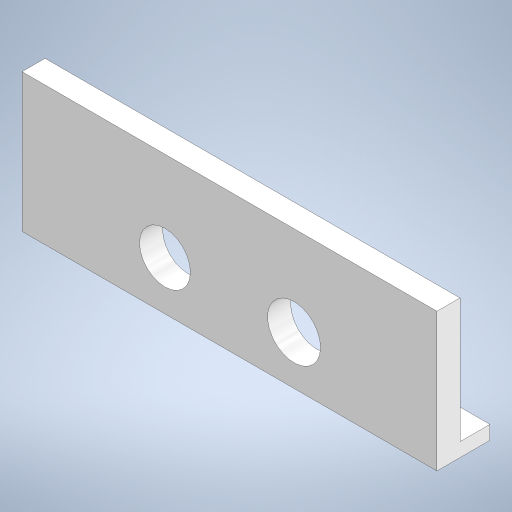
# Autodesk Inventor part: wall
Saved by Autodesk Inventor 2024 (Build 280153000, 153)
## iProperties
Created: 2023-08-11
Part Number: wall
Material: ABS Plastic
Document SubType Name: Modeling
Designer: l1534
Density: 1.06 g/cm^3
Appearance: Smooth - White
Author: l1534
Autodesk Inventor part; units mm, degrees
ref_plane "YZ Plane" through (0, 0, 0) normal (1, 0, 0) x (0, 1, 0)
ref_plane "XZ Plane" through (0, 0, 0) normal (0, 1, 0) x (-1, 0, 0)
ref_plane "XY Plane" through (0, 0, 0) normal (0, 0, 1) x (1, 0, 0)
sketch "Sketch1" plane through (0, 0, 0) normal (0, 0, 1) x (1, 0, 0)
  line L0 (-96.9802, 31.1578) -> (83.0198, 31.1578)
  line L1 (83.0198, 31.1578) -> (83.0198, -28.8422)
  line L2 (83.0198, -28.8422) -> (-96.9802, -28.8422)
  line L3 (-96.9802, -28.8422) -> (-96.9802, 31.1578)
  point P0 (0, 0)
  dimension "d0" = 180
  dimension "d1" = 60
  constraints: 8 end point, 2 parallel, 1 horizontal, 1 perpendicular
  measures "d0" distance of L0.start L0.end
  measures "d1" distance of L0.end L1.end
extrude "Extrusion1" add sketch "Sketch1" along normal blind 10
sketch "Sketch4" plane through (0, 0, 0) normal (0, 0, -1) x (-1, 0, 0)
  circle A0 centre (-21.0198, -7.6922) radius 11.5
  line L0 (96.9802, -28.8422) -> (-83.0198, -28.8422) projected
  line L1 (-83.0198, -28.8422) -> (-83.0198, 31.1578) projected
  point P0 (0, 0)
  dimension "d16" = 23
  dimension "d17" = 21.15
  dimension "d18" = 62
  constraints: 1 centre point
  measures "d16" diameter of A0
  measures "d17" distance from line of L0 A0.centre
  measures "d18" distance from line of L1 A0.centre
extrude "Extrusion4" cut sketch "Sketch4" against normal through all
sketch "Sketch5" plane through (0, 0, 0) normal (0, 0, -1) x (-1, 0, 0)
  line L0 (96.9802, -28.8422) -> (-83.0198, -28.8422) projected
  line L1 (96.9802, 31.1578) -> (96.9802, -28.8422) projected
  line L2 (-83.0198, -28.8422) -> (96.9802, -28.8422)
  line L3 (96.9802, -28.8422) -> (96.9802, -22.8422)
  line L4 (96.9802, -22.8422) -> (-83.0198, -22.8422)
  line L5 (-83.0198, -22.8422) -> (-83.0198, -28.8422)
  point P0 (0, 0)
  dimension "d21" = 6
  constraints: 8 end point, 2 parallel, 1 horizontal, 1 perpendicular, 1 point on line
  measures "d21" distance between parallel lines of L0 L4
extrude "Extrusion5" add sketch "Sketch5" along normal blind 13
sketch "Sketch6" plane through (-96.9802, -22.8422, 0) normal (0, 1, 0) x (1, 0, 0)
  line L0 (180, 13) -> (0, 13) projected
  line L1 (180, 0) -> (0, 0) projected
  line L2 (159.9, 13) -> (153.9, 13)
  line L3 (153.9, 13) -> (153.9, 0)
  line L4 (153.9, 0) -> (159.9, 0)
  line L5 (159.9, 0) -> (159.9, 13)
  line L6 (20.1, 13) -> (26.1, 13)
  line L7 (26.1, 13) -> (26.1, 0)
  line L8 (26.1, 0) -> (20.1, 0)
  line L9 (20.1, 0) -> (20.1, 13)
  line L10 (0, 0) -> (0, 13) projected
  line L11 (180, 0) -> (180, 13) projected
  point P0 (96.9802, 0)
  point P1 (20.1, 13)
  point P2 (20.1, 0)
  point P3 (26.1, 13)
  dimension "d24" = 20.1
  dimension "d25" = 6
  dimension "d26" = 20.1
  dimension "d27" = 6
  constraints: 16 end point, 4 parallel, 4 point on line, 2 horizontal, 2 perpendicular
  measures "d24" distance between parallel lines of L10 L9
  measures "d25" distance between parallel lines of L7 L9
  measures "d26" distance between parallel lines of L11 L5
  measures "d27" distance between parallel lines of L5 L3
extrude "Extrusion6" add sketch "Sketch6" along normal blind 20 contours L5 L1 L3 L0 | L7 L1 L9 L0
sketch "Sketch7" plane through (-70.8802, -22.8422, 0) normal (0, 1, 0) x (1, 0, 0)
  line L0 (0, 13) -> (127.8, 13) projected
  line L1 (0, 13) -> (0, 0) projected
  line L2 (127.8, 13) -> (0, 13)
  line L3 (0, 13) -> (0, 0)
  line L4 (0, 0) -> (127.8, 0)
  line L5 (127.8, 0) -> (127.8, 13)
  point P0 (70.8802, 0)
  constraints: 8 end point, 2 parallel, 1 horizontal, 1 perpendicular
extrude "Extrusion7" cut sketch "Sketch7" against normal through all
chamfer "Chamfer1" distance 3 angle 45 2 edges at (56.9198, -28.8422, -6.5) (-70.8802, -28.8422, -6.5)
sketch "Sketch8" plane through (0, 0, 10) normal (0, 0, 1) x (1, 0, 0)
  circle A0 centre (-34.9802, -7.6922) radius 11.05
  line L0 (-96.9802, -28.8422) -> (83.0198, -28.8422) projected
  line L1 (-96.9802, 31.1578) -> (-96.9802, -28.8422) projected
  point P0 (0, 0)
  dimension "d35" = 22.1
  dimension "d36" = 21.15
  dimension "d37" = 62
  constraints: 1 centre point
  measures "d35" diameter of A0
  measures "d36" distance from line of L0 A0.centre
  measures "d37" distance from line of L1 A0.centre
extrude "Extrusion8" cut sketch "Sketch8" against normal through all
body "Solid1"
